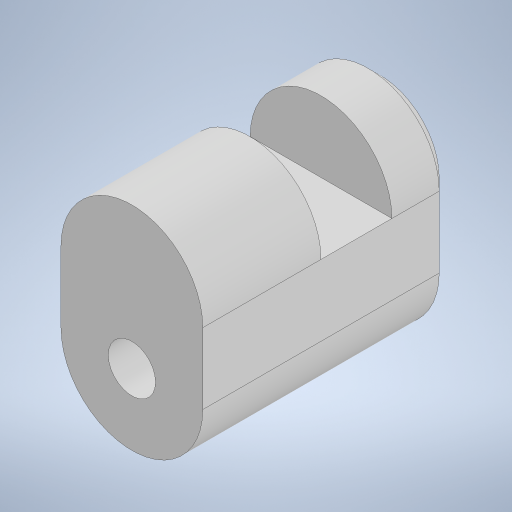
# Autodesk Inventor part: picture-fixings-8mm
Saved by Autodesk Inventor 2024.1 (Build 281209000, 209)
## iProperties
Created: 2025-09-26
Part Number: picture-fixings-8mm
Material: Generic
Document SubType Name: Modeling
Designer: iwheard
Density: 1 g/cm^3
Appearance: Default
Author: iwheard
Autodesk Inventor part; units mm, degrees
ref_plane "YZ Plane" through (0, 0, 0) normal (1, 0, 0) x (0, 1, 0)
ref_plane "XZ Plane" through (0, 0, 0) normal (0, 1, 0) x (-1, 0, 0)
ref_plane "XY Plane" through (0, 0, 0) normal (0, 0, 1) x (1, 0, 0)
sketch "Sketch2" plane through (0, 0, 0) normal (0, 0, 1) x (1, 0, 0)
  circle A0 centre (0, 0) radius 6
  circle A1 centre (0, 0) radius 2
  dimension "d0" = 12
  dimension "d1" = 4
  constraints: 2 centre point, 1 concentric
  measures "d0" diameter of A0
  measures "d1" diameter of A1
extrude "Extrusion1" add sketch "Sketch2" along normal blind 21
sketch "Sketch3" plane through (0, 0, 21) normal (0, 0, 1) x (1, 0, 0)
  line L0 (0, 0) -> (0, 6) construction
  line L1 (6, 0) -> (6, 6)
  line L2 (-6, 6) -> (-6, 0)
  arc A0 (-6, 0) -> (6, 0) centre (0, 0) ccw
  arc A1 (6, 6) -> (-6, 6) centre (0, 6) ccw
  circle A2 centre (0, 0) radius 2 projected
  circle A3 centre (0, 0) radius 6 projected
  circle A4 centre (0, 0) radius 2 projected
  circle A5 centre (0, 0) radius 6 projected
  point P0 (0, 3)
  dimension "d4" = 6
  dimension "d5" = 6
  constraints: 8 end point, 4 point on circle, 4 tangent, 2 centre point, 1 concentric, 1 midpoint, 1 parallel
  measures "d4" radius of A0
  measures "d5" distance of L0.end point (0, 0)
extrude "Extrusion2" add sketch "Sketch3" against normal blind 10 contours A3 L2 A1 L1
sketch "Sketch4" plane through (0, 0, 0) normal (0, 0, -1) x (-1, 0, 0)
  arc A0 (6, 6) -> (-6, 6) centre (0, 6) ccw projected
  line L0 (-6, 6) -> (-6, 0) projected
  line L1 (6, 0) -> (6, 6) projected
  arc A1 (6, 0) -> (-6, 0) centre (0, 0) ccw projected
  circle A2 centre (0, 0) radius 2 projected
extrude "Extrusion3" add sketch "Sketch4" against normal blind 5 contours L1 A1 L0 A0
sketch "Sketch5" plane through (0, 0, 11) normal (0, 0, -1) x (-1, 0, 0)
  arc A0 (6, 6) -> (-6, 6) centre (0, 6) ccw projected
  line L0 (-6, 6) -> (-6, 0) projected
  line L1 (6, 0) -> (6, 6) projected
  arc A1 (6, 0) -> (-6, 0) centre (0, 0) ccw projected
  line L2 (-6, 6) -> (6, 6)
  arc A2 (6, 0) -> (-6, 0) centre (0, 0) ccw projected
  point P0 (0, 6)
  constraints: 2 end point, 2 point on line, 1 horizontal alignment, 1 tangent
extrude "Extrusion4" add sketch "Sketch5" along normal blind 6.4 contours L1 A1 L2 | L2 A1 L0
chamfer "Chamfer1" distance 3 angle 45 1 edges at (-2, 0, 0)
chamfer "Chamfer2" distance 1 angle 45 3 edges at (-6, 3, 0) (0, 12, 0) (6, 3, 0)
body "Solid1"
